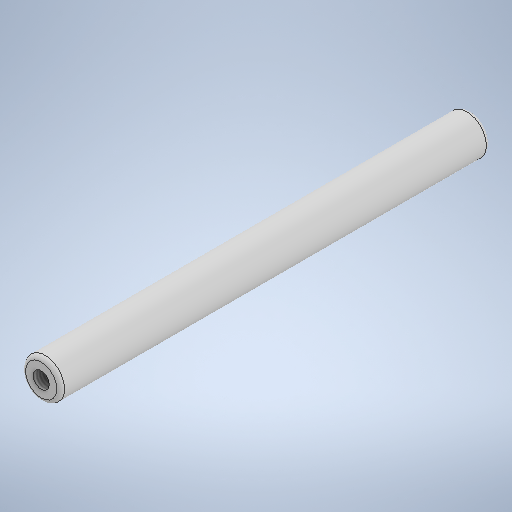
# Autodesk Inventor part: 121
Saved by Autodesk Inventor 2025.1 (Build 291241000, 241)
## iProperties
Created: 2024-08-05
Part Number: 121
Material: Generisch
Document SubType Name: Modeling
Designer: ffogue
Density: 1 g/cm^3
Appearance: Vorgabe
Author: ffogue
Autodesk Inventor part; units mm, degrees
ref_plane "YZ Plane" through (0, 0, 0) normal (1, 0, 0) x (0, 1, 0)
ref_plane "XZ Plane" through (0, 0, 0) normal (0, 1, 0) x (-1, 0, 0)
ref_plane "XY Plane" through (0, 0, 0) normal (0, 0, 1) x (1, 0, 0)
sketch "Sketch1" plane through (0, 0, 0) normal (0, 0, 1) x (1, 0, 0)
  line L0 (0, 0) -> (0, 110)
  line L1 (0, 110) -> (5, 110)
  line L2 (5, 110) -> (5, 0)
  line L3 (5, 0) -> (0, 0)
  dimension "d0" = 110
  dimension "d1" = 10
  constraints: 8 end point, 3 perpendicular, 1 vertical
  measures "d0" distance of L0.start L0.end
  measures "d1" diameter of L2 L0
revolve "Revolution1" add sketch "Sketch1" angle 360 about axis through (0, 0, 0) along (0, 1, 0)
fillet "Fillet1" radius 1 2 edges at (-5, 0, 0) (-5, 110, 0)
sketch "Sketch2" plane through (0, 110, 0) normal (0, 1, 0) x (1, 0, 0)
  circle A0 centre (0, 0) radius 5 projected
  constraints: 1 coincident
hole "Hole1" at (0, 110, 0) direction (0, -1, 0) diameter 4.134 depth 12 thread size "M5x0.8" class "6H" standard "ISO Metric profile"
sketch "Sketch3" plane through (0, 0, 0) normal (0, -1, 0) x (1, 0, 0)
  circle A0 centre (0, 0) radius 5 projected
  constraints: 1 coincident
hole "Hole2" at (0, 0, 0) direction (0, 1, 0) diameter 4.134 depth 12 thread size "M5x0.8" class "6H" standard "ISO Metric profile"
body "Solid1"
